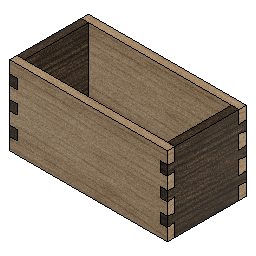
dovetail_box (Autodesk Fusion 360 design; units mm, degrees)
Autodesk Fusion 360 part; units mm, degrees
sketch "Sketch1" plane through (0, 0, 0) normal (0, 1, 0) x (1, 0, 0)
  line L0 (0, 0) -> (101.6, 0)
  line L1 (101.6, 0) -> (101.6, -101.6)
  line L2 (101.6, -101.6) -> (0, -101.6)
  line L3 (0, -101.6) -> (0, 0)
  line L4 (9.525, -101.6) -> (9.525, 0) construction
  line L5 (92.075, -101.6) -> (92.075, 0) construction
  line L6 (92.075, -85.725) -> (101.6, -85.725)
  line L7 (92.075, -85.725) -> (101.6, -85.725)
  line L8 (101.6, -85.725) -> (101.6, -73.025)
  line L9 (101.6, -73.025) -> (92.075, -73.025)
  line L10 (92.075, -73.025) -> (92.075, -85.725)
  line L11 (101.6, -44.45) -> (92.075, -44.45)
  line L12 (92.075, -44.45) -> (92.075, -57.15)
  line L13 (92.075, -57.15) -> (101.6, -57.15)
  line L14 (101.6, -15.875) -> (92.075, -15.875)
  line L15 (92.075, -15.875) -> (92.075, -28.575)
  line L16 (92.075, -28.575) -> (101.6, -28.575)
  dimension "d8" = 101.6
  dimension "d9" = 101.6
  dimension "d10" = 9.525
  dimension "d12" = 9.525
  dimension "d19" = 15.875
  dimension "d20" = 12.7
  dimension "d23" = 0
  dimension "d24" = 28.575
  constraint horizontal L0
  constraint vertical L1
  constraint horizontal L2
  constraint vertical L3
  constraint coincident L0.start L3.end
  constraint coincident L2 L4.start
  constraint coincident L0 L4.end
  constraint perpendicular L0 L4
  constraint coincident L2 L5.start
  constraint coincident L0 L5.end
  constraint perpendicular L0 L5
  constraint coincident L5 L6.start
  constraint coincident L1 L6.end
  constraint perpendicular L1 L6
  constraint horizontal L7
  constraint vertical L8
  constraint horizontal L9
  constraint vertical L10
  constraint collinear L1 L8
  measures "d8" distance of L0.start L0.end
  measures "d9" distance of L0.start L2.end
  measures "d10" distance of L3 L4
  measures "d12" distance of L1 L5
  measures "d19" distance of L2 L6
  measures "d20" distance of L6.start L9.end
extrude "Extrude1" add sketch "Sketch1" along normal blind 9.525 makes body 1
sketch "Sketch2" plane through (101.6, 0, 0) normal (1, 0, 0) x (0, 1, 0)
  line L0 (0, 101.6) -> (0, 0)
  line L1 (0, 0) -> (9.525, 0)
  line L2 (9.525, 0) -> (9.525, 101.6)
  line L3 (9.525, 101.6) -> (0, 101.6)
  line L4 (0, 85.725) -> (9.525, 84.5335)
  line L5 (0, 85.725) -> (12.799, 85.725) construction
  line L6 (0, 57.15) -> (9.525, 55.9585)
  line L7 (0, 73.025) -> (9.525, 74.2165)
  line L8 (0, 73.025) -> (12.799, 73.025) construction
  line L9 (0, 44.45) -> (9.525, 45.6415)
  line L10 (0, 28.575) -> (9.525, 27.3835)
  line L11 (0, 15.875) -> (9.525, 17.0665)
  point P0 (0, 85.725)
  point P1 (0, 73.025)
  dimension "d26" = 7.13
  dimension "d29" = 0
  dimension "d31" = 7.13
  dimension "d34" = 0
  constraint horizontal L5
  constraint coincident P0 L4.start
  constraint coincident L2 L4.end
  constraint horizontal L8
  constraint coincident P1 L7.start
  constraint coincident L2 L7.end
  measures "d26" angle of L4 L5
  measures "d31" angle of L7 L8
sketch "Sketch3" plane through (101.6, 0, 0) normal (1, 0, 0) x (0, 1, 0)
sketch "Sketch4" plane through (101.6, 0, 0) normal (1, 0, 0) x (0, 1, 0)
  line L0 (0, 101.6) -> (50.8, 101.6)
  line L1 (50.8, 101.6) -> (50.8, 0)
  line L2 (50.8, 0) -> (0, 0)
  line L3 (0, 0) -> (0, 101.6)
  point P0 (0, 101.6)
  dimension "d36" = 50.8
  dimension "d37" = 101.6
  constraint horizontal L0
  constraint vertical L1
  constraint horizontal L2
  constraint vertical L3
  constraint coincident P0 L0.start
  measures "d36" distance of P0 L0.end
  measures "d37" distance of P0 L2.end
extrude "Extrude2" add sketch "Sketch4" against normal blind 9.525 separate body makes body 2
extrude "Extrude3" cut sketch "Sketch2" against normal blind 9.525 contours L0 L2 L3 L4 bodies 2
ref_plane "WorkPlane1" through (50.8, 4.7625, 50.8) normal (0, 0, 1) x (1, 0, 0)
mirror "Mirror1" about plane through (50.8, 4.7625, 50.8) normal (0, 0, 1) of "Extrude3"
extrude "Extrude4" cut sketch "Sketch2" against normal blind 9.525 contours L0 L2 L6 L7 bodies 2
pattern_linear "R-Pattern1" count 2 spacing 28.575 along (0, 0, -1) of "Extrude4"
extrude "Extrude5" cut sketch "Sketch2" against normal blind 9.525 contours L0 L2 L4 L7 bodies 1
pattern_linear "R-Pattern2" count 3 spacing 28.575 along (0, 0, -1) of "Extrude5"
mirror "Mirror2" about plane through (101.6, 50.8, 101.6) normal (0, 1, 0) of bodies 2 merged
mirror "Mirror3" about plane through (0, 0, 101.6) normal (-1, 0, 0) of bodies 1 merged
mirror "Mirror4" about plane through (0, 9.525, 0) normal (0, 1, 0) of bodies 1 makes body 3
move_body "Move1" bodies 3 to x (1, 0, 0) y (0, 1, 0) z (0, 0, 1) at (0, 82.55, 0)
copy_body "CopyPasteBodies1" bodies 2 makes body 4
move_body "Move2" bodies 4 to x (1, 0, 0) y (0, 1, 0) z (0, 0, 1) at (-193.675, 0, 0)
copy_body "Body->Comp1" bodies 4 removing the originals makes body 5 in component "left"
copy_body "Body->Comp2" bodies 3 removing the originals makes body 6 in component "back"
copy_body "Body->Comp3" bodies 2 removing the originals makes body 7 in component "right"
copy_body "Body->Comp4" bodies 1 removing the originals makes body 8 in component "front"
component "left" placed x (1, 0, 0) y (0, 1, 0) z (0, 0, 1) at (0, 0, 0)
component "back" placed x (1, 0, 0) y (0, 1, 0) z (0, 0, 1) at (0, 0, 0)
component "right" placed x (1, 0, 0) y (0, 1, 0) z (0, 0, 1) at (0, 0, 0)
component "front" placed x (1, 0, 0) y (0, 1, 0) z (0, 0, 1) at (0, 0, 0)
equation "WallHeight = 4 in"
equation "FrontLength = 8 in"
equation "FrontThickness = ( 3 / 8 ) * 1 in"
equation "SideLength = 4 in"
equation "SideThickness = ( 3 / 8 ) * 1 in"
equation "d8 = FrontLength / 2"
equation "d9 = WallHeight"
equation "d10 = SideThickness + DovetailPride"
equation "DovetailPride = 0 in"
equation "d12 = SideThickness + DovetailPride"
equation "PinCount = 3"
equation "d14 = FrontThickness"
equation "PinWidth = 0.5 in"
equation "PinSpacing = ( WallHeight - ( PinCount * PinWidth ) ) / ( PinCount + 1 )"
equation "d19 = PinSpacing"
equation "d20 = PinWidth"
equation "d22 = PinCount"
equation "d24 = PinSpacing + PinWidth"
equation "TailAngle = 7.13 deg"
equation "d26 = TailAngle"
equation "d28 = PinCount"
equation "d30 = -PinWidth - PinSpacing"
equation "d31 = TailAngle"
equation "d33 = PinCount"
equation "d35 = -PinWidth - PinSpacing"
equation "d36 = SideLength / 2"
equation "d37 = WallHeight"
equation "d38 = -SideThickness"
equation "d40 = -SideThickness"
equation "d42 = -WallHeight / 2"
equation "d45 = -SideThickness"
equation "d47 = PinCount - 1"
equation "d49 = PinSpacing + PinWidth"
equation "d51 = -SideThickness"
equation "d53 = PinCount"
equation "d55 = PinWidth + PinSpacing"
equation "d64 = SideLength - FrontThickness * 2"
equation "d66 = -FrontLength + SideThickness"
named bodies: "front", "right", "back", "left"
